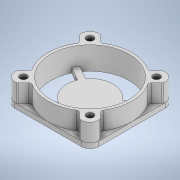
# Autodesk Inventor part: SmallFanCase
Saved by Autodesk Inventor 2022 (Build 260153000, 153)
## iProperties
Created: 2023-05-17
Part Number: SmallFanCase
Material: Generic
Document SubType Name: Modeling
Designer: richb366163
Density: 1 g/cm^3
Appearance: Default
Author: richb366163
Autodesk Inventor part; units mm, degrees
ref_plane "YZ Plane" through (0, 0, 0) normal (1, 0, 0) x (0, 1, 0)
ref_plane "XZ Plane" through (0, 0, 0) normal (0, 1, 0) x (-1, 0, 0)
ref_plane "XY Plane" through (0, 0, 0) normal (0, 0, 1) x (1, 0, 0)
sketch "Sketch1" plane through (0, 0, 0) normal (0, 1, 0) x (-1, 0, 0)
  line L0 (4.318, 0) -> (36.195, 0)
  line L1 (40.513, -4.318) -> (40.513, -36.195)
  line L2 (36.195, -40.513) -> (4.318, -40.513)
  line L3 (0, -36.195) -> (0, -4.318)
  circle A0 centre (20.2565, -20.2565) radius 18.923
  arc A1 (40.513, -4.318) -> (36.195, 0) centre (36.195, -4.318) ccw
  arc A2 (36.195, -40.513) -> (40.513, -36.195) centre (36.195, -36.195) ccw
  arc A3 (0, -36.195) -> (4.318, -40.513) centre (4.318, -36.195) ccw
  arc A4 (4.318, 0) -> (0, -4.318) centre (4.318, -4.318) ccw
  circle A5 centre (20.2565, -20.2565) radius 11.176
  line L4 (20.2565, -9.0805) -> (20.2565, -1.3335)
  line L5 (21.6535, -9.0805) -> (21.6535, -1.3335)
  line L6 (18.8595, -9.0805) -> (18.8595, -1.3335)
  line L7 (21.6535, -9.0805) -> (21.6535, -9.9558)
  line L8 (18.8595, -9.0805) -> (18.8595, -9.7427)
  line L9 (9.8793, -24.6347) -> (3.1702, -28.5082)
  line L10 (9.8793, -24.6347) -> (10.6373, -24.197)
  line L11 (11.2763, -27.0543) -> (4.5672, -30.9278)
  line L12 (11.2763, -27.0543) -> (11.8497, -26.7233)
  line L13 (29.2367, -27.0543) -> (35.9458, -30.9278)
  line L14 (29.2367, -27.0543) -> (28.4787, -26.6167)
  line L15 (30.6337, -24.6347) -> (37.3428, -28.5082)
  line L16 (30.6337, -24.6347) -> (30.0603, -24.3036)
  line L17 (20.2565, -20.2565) -> (34.6075, -20.2565)
  line L18 (34.6075, -20.2565) -> (34.6075, -5.9055)
  line L19 (34.6075, -5.9055) -> (20.2565, -5.9055)
  line L20 (20.2565, -5.9055) -> (20.2565, -20.2565)
  line L21 (34.6075, -5.9055) -> (38.0365, -5.9055)
  line L22 (38.0365, -5.9055) -> (38.0365, -2.4765)
  line L23 (38.0365, -2.4765) -> (34.6075, -2.4765)
  line L24 (34.6075, -2.4765) -> (34.6075, -5.9055)
  circle A6 centre (36.322, -4.191) radius 1.7145
  circle A7 centre (4.191, -4.191) radius 1.7145
  circle A8 centre (36.322, -36.322) radius 1.7145
  circle A9 centre (4.191, -36.322) radius 1.7145
  point P0 (0, 0)
  point P1 (40.513, -40.513)
  point P2 (40.513, 0)
  point P3 (0, -40.513)
  point P4 (21.6535, -9.1682)
  point P5 (21.6535, -1.3851)
  point P6 (37.2981, -28.4823)
  point P7 (30.5578, -24.5908)
  point P8 (18.8595, -9.1682)
  point P9 (9.9552, -24.5908)
  point P10 (3.2149, -28.4823)
  point P11 (18.8595, -1.3851)
  point P12 (11.3522, -27.0105)
  point P13 (29.1608, -27.0105)
  point P14 (35.9011, -30.902)
  point P15 (4.6119, -30.902)
  dimension "d2" = 37.846
  dimension "d4" = 22.352
  dimension "d0" = 40.513
  dimension "d1" = 40.513
  dimension "d3" = 4.318
  dimension "d5" = 1.397
  dimension "d6" = 1.397
  dimension "d9" = 360
  dimension "d25" = 14.351
  dimension "d26" = 14.351
  dimension "d27" = 3.429
  dimension "d28" = 3.429
  constraints: 50 end point, 8 centre point, 8 parallel, 8 point on circle, 8 point on line, 8 tangent, 3 equal radius, 3 horizontal, 3 perpendicular, 3 symmetric about line, 3 vertical, 1 coincident, 40 other
  measures "d0" distance of point (40.513, -40.513) point (0, -40.513)
  measures "d1" distance of point (40.513, 0) point (40.513, -40.513)
  measures "d3" radius of A1
  measures "d5" distance between parallel lines of L4 L5
  measures "d6" distance between parallel lines of L4 L6
  measures "d25" distance of L19.end L18.end
  measures "d26" distance of L18.end L17.end
  measures "d27" distance of L23.end L22.end
  measures "d28" distance of L22.end L21.end
extrude "Extrusion1" add sketch "Sketch1" along normal blind 2.413 contours L0 A1 L1 A2 L2 A3 L3 A4 | L24 A6 L21 | A0 L19 L18 | A0 L13 L14 A5 L16 L15 | L5 L19 L4 A0 | L5 L7 A5 L4 L19 | L17 L20 A5 | A5 L20 L17 | A6 L22 L21 | L24 L23 A6 | A0 L9 L10 A5 L12 L11 | L4 A5 L8 L6 A0 | A6 L23 L22
sketch "Sketch2" plane through (0, 2.413, 0) normal (0, 1, 0) x (1, 0, 0)
  arc A0 (-18.8595, 1.3851) -> (-3.2149, 28.4823) centre (-20.2565, 20.2565) ccw projected
  circle A1 centre (-20.2565, 20.2565) radius 20.2565
  arc A2 (-4.6119, 30.902) -> (-35.9011, 30.902) centre (-20.2565, 20.2565) ccw projected
  circle A3 centre (-20.2565, 20.2565) radius 18.923
  line L0 (-20.2565, 20.2565) -> (-20.2565, 10.2449)
  line L1 (-20.2565, 20.2565) -> (-12.0868, 20.2565)
  circle A4 centre (-4.191, 36.322) radius 1.7145 projected
  circle A5 centre (-4.191, 36.322) radius 1.7145
  circle A6 centre (-4.191, 36.322) radius 4.1384
  line L2 (-0.1946, 35.2471) -> (-5.4682, 29.9735)
  line L3 (-0.1946, 35.2471) -> (7.2634, 35.2471) construction
  line L4 (-4.191, 36.322) -> (-0.4031, 40.1099)
  line L5 (-5.2659, 40.3184) -> (-10.5395, 35.0448)
  line L6 (-40.3184, 35.2471) -> (-35.0448, 29.9735)
  circle A7 centre (-36.322, 36.322) radius 4.1384
  circle A8 centre (-36.322, 36.322) radius 1.7145
  line L7 (-35.2471, 40.3184) -> (-29.9735, 35.0448)
  line L8 (-35.2471, 0.1946) -> (-29.9735, 5.4682)
  circle A9 centre (-36.322, 4.191) radius 4.1384
  circle A10 centre (-36.322, 4.191) radius 1.7145
  line L9 (-40.3184, 5.2659) -> (-35.0448, 10.5395)
  line L10 (-0.1946, 5.2659) -> (-5.4682, 10.5395)
  circle A11 centre (-4.191, 4.191) radius 4.1384
  circle A12 centre (-4.191, 4.191) radius 1.7145
  line L11 (-5.2659, 0.1946) -> (-10.5395, 5.4682)
  point P0 (-3.2149, 28.4823)
  point P1 (-18.8595, 1.3851)
  point P2 (-31.8181, 3.6236)
  point P3 (-36.8894, 8.6949)
  point P4 (-8.6949, 3.6236)
  point P5 (-3.6236, 8.6949)
  point P6 (-8.6949, 36.8894)
  point P7 (-3.6236, 31.8181)
  point P8 (-36.8894, 31.8181)
  point P9 (-31.8181, 36.8894)
  dimension "d29" = 135
  dimension "d32" = 360
  constraints: 24 end point, 7 coincident, 5 centre point, 2 horizontal, 2 symmetric about line, 1 equal length, 1 vertical, 56 other
  measures "d29" angle of L2 L3
extrude "Extrusion2" add sketch "Sketch2" along normal blind 8.636 contours A0 A3 L2 A1 L10 | L10 A1 A11 A0 | A3 A2 A6 A1 L2 | A11 A1 A0 | L10 A11 A1 | A1 A6 L2 | A11 A1 L11 A0 | A11 L10 L11 A1 | A2 A6 A1 | A1 A6 L5 L2 | L11 A1 L8 A3 A0 | A11 L11 A1 | A2 L5 A1 A6 | A1 L5 A6 | A2 L7 A1 L5 | L8 A1 A9 A3 | L8 A9 A1 | A2 A7 A1 L7 | A1 A7 L7 | A9 A1 A3 | A9 L8 L9 A1 | A2 A7 A1 | A1 A7 L6 L7 | A9 A1 L9 A3 | A9 L9 A1 | A2 A3 L6 A1 A7 | A1 L6 A7 | L9 A1 L6 A3
fillet "Fillet2" radius 1.27 16 edges at (-35.2471, 6.731, -0.1946) (-31.8181, 6.731, -3.6236) (-8.6949, 6.731, -36.8894) (-3.6236, 6.731, -31.8181) (-5.2659, 6.731, -40.3184) (-0.1946, 6.731, -35.2471) (-5.2659, 6.731, -0.1946) (-8.6949, 6.731, -3.6236) (-0.1946, 6.731, -5.2659) (-3.6236, 6.731, -8.6949) (-36.8894, 6.731, -8.6949) (-40.3184, 6.731, -5.2659) (-35.2471, 6.731, -40.3184) (-31.8181, 6.731, -36.8894) (-36.8894, 6.731, -31.8181) (-40.3184, 6.731, -35.2471)
body "Solid1"
